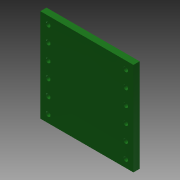
# Autodesk Inventor part: Board
Saved by Autodesk Inventor 2013 (Build 170138000, 138)
## iProperties
Created: 2013-07-31
Part Number: Board
Material: Thermoplastic Resin
Document SubType Name: Modeling
Designer: Kyle
Density: 1 g/cm^3
Author: Kyle
Autodesk Inventor part; units mm, degrees
ref_plane "YZ Plane" through (0, 0, 0) normal (1, 0, 0) x (0, 1, 0)
ref_plane "XZ Plane" through (0, 0, 0) normal (0, 1, 0) x (-1, 0, 0)
ref_plane "XY Plane" through (0, 0, 0) normal (0, 0, 1) x (1, 0, 0)
sketch "Sketch1" plane through (0, 0, 0) normal (0, 0, 1) x (1, 0, 0)
  line L0 (0, 0) -> (15.24, 0)
  line L1 (15.24, 0) -> (15.24, -15.24)
  line L2 (15.24, -15.24) -> (0, -15.24)
  line L3 (0, -15.24) -> (0, 0)
  dimension "d0" = 15.24
  dimension "d1" = 15.24
  constraints: 8 end point, 2 parallel, 1 horizontal, 1 perpendicular
  measures "d0" distance of L0.start L0.end
  measures "d1" distance of L0.end L1.end
extrude "Extrusion1" add sketch "Sketch1" along normal blind 1.016
sketch "Sketch2" plane through (0, 0, 1.016) normal (0, 0, 1) x (1, 0, 0)
  line L0 (15.24, 0) -> (0, 0) projected
  line L1 (0, 0) -> (0, -15.24) projected
  line L2 (15.24, -15.24) -> (15.24, 0) projected
  circle A0 centre (13.97, -1.27) radius 0.381
  circle A1 centre (13.97, -3.81) radius 0.381
  circle A2 centre (13.97, -6.35) radius 0.381
  circle A3 centre (13.97, -8.89) radius 0.381
  circle A4 centre (13.97, -11.43) radius 0.381
  circle A5 centre (13.97, -13.97) radius 0.381
  circle A6 centre (1.27, -1.27) radius 0.381
  circle A7 centre (1.27, -3.81) radius 0.381
  circle A8 centre (1.27, -6.35) radius 0.381
  circle A9 centre (1.27, -8.89) radius 0.381
  circle A10 centre (1.27, -11.43) radius 0.381
  circle A11 centre (1.27, -13.97) radius 0.381
  dimension "d4" = 0.762
  dimension "d6" = 1.27
  dimension "d7" = 1.27
  dimension "d10" = 2.54
  dimension "d17" = 12.7
  constraints: 12 centre point, 1 horizontal, 1 vertical, 22 other
  measures "d4" diameter of A0
  measures "d6" distance from line of L0 A0.centre
  measures "d7" distance from line of L2 A0.centre
  measures "d10" distance of A0.centre A1.centre
  measures "d17" distance of A0.centre A6.centre
extrude "Extrusion2" cut sketch "Sketch2" against normal blind 1.27
body "Solid1"
